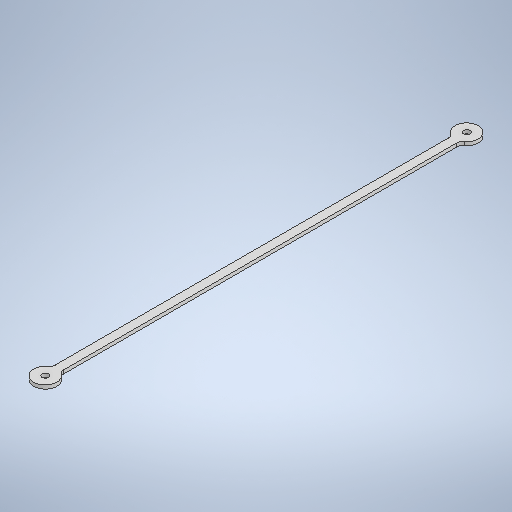
# Autodesk Inventor part: A2P3
Saved by Autodesk Inventor 2025.2 (Build 292293000, 293)
## iProperties
Created: 2025-05-22
Part Number: A2P3
Material: Generic
Document SubType Name: Sheet Metal
Designer: Admin
Density: 1 g/cm^3
Sheet Metal Rule: Default
Appearance: Default
Author: Admin
Autodesk Inventor part; units mm, degrees
ref_plane "YZ Plane" through (0, 0, 0) normal (1, 0, 0) x (0, 1, 0)
ref_plane "XZ Plane" through (0, 0, 0) normal (0, 1, 0) x (-1, 0, 0)
ref_plane "XY Plane" through (0, 0, 0) normal (0, 0, 1) x (1, 0, 0)
sketch "Sketch1" plane through (0, 0, 0) normal (0, 1, 0) x (-1, 0, 0)
  arc A0 (3.17, -4.4332) -> (-3.17, -4.4332) centre (0, 0) ccw
  line L0 (2, -6.7082) -> (2, -193.2918)
  line L1 (-2, -6.7082) -> (-2, -193.2918)
  arc A1 (3.17, -4.4332) -> (2, -6.7082) centre (4.7967, -6.7082) ccw
  arc A2 (-2, -6.7082) -> (-3.17, -4.4332) centre (-4.7967, -6.7082) ccw
  arc A3 (-3.17, -195.5668) -> (3.17, -195.5668) centre (0, -200) ccw
  arc A4 (2, -193.2918) -> (3.17, -195.5668) centre (4.7967, -193.2918) ccw
  arc A5 (-3.17, -195.5668) -> (-2, -193.2918) centre (-4.7967, -193.2918) ccw
  dimension "d0" = 10.9
  dimension "d2" = 4
  dimension "d3" = 2
  dimension "d4" = 10.9
  dimension "d5" = 2
  dimension "d6" = 0
  dimension "d7" = 200
  dimension "d8" = 7
  dimension "d9" = 7
  dimension "d10" = 0
  constraints: 12 point on circle, 8 tangent, 6 centre point, 4 end point, 2 vertical, 1 coincident
  measures "d0" diameter of A0
  measures "d2" horizontal distance of L1.end L0.start
  measures "d3" horizontal distance of L0.start point (0, 0)
  measures "d4" diameter of A3
  measures "d5" horizontal distance of L0.end A3.centre
  measures "d6" vertical distance of L1.end L0.end
  measures "d7" distance of point (0, 0) A3.centre
  measures "d8" distance of point (0, 0) L0.start
  measures "d9" distance of A3.centre L0.end
  measures "d10" vertical distance of L1.start L0.start
extrude "Extrusion1" add sketch "Sketch1" along normal blind 1.7
sketch "Sketch2" plane through (0, 1.7, 0) normal (0, 1, 0) x (1, 0, 0)
  circle A0 centre (0, 0) radius 1.5
  arc A1 (3.17, 195.5668) -> (-3.17, 195.5668) centre (0, 200) ccw projected
  circle A2 centre (0, 200) radius 1.5
  dimension "d13" = 3
  dimension "d14" = 3
  constraints: 2 centre point, 2 coincident
  measures "d13" diameter of A0
  measures "d14" diameter of A2
extrude "Extrusion2" cut sketch "Sketch2" against normal blind 1.7
equation "\"BendRadius\" = Thickness"
equation "\"BendReliefWidth\" = Thickness"
equation "\"BendReliefDepth\" = 0.5 * Thickness"
equation "\"CornerReliefSize\" = 4 * Thickness"
equation "\"MinimumRemnant\" = 2 * Thickness"
equation "\"TransitionRadius\" = BendRadius"
equation "\"JacobiRadiusSize\" = BendRadius"
equation "\"GapSize\" = Thickness"
equation "\"Thickness\" = 3.048"
body "Solid1"
